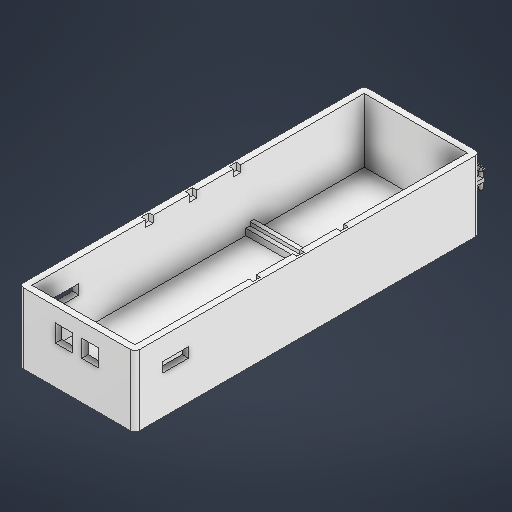
# Autodesk Inventor part: module_switch
Saved by Autodesk Inventor 2025.4 (Build 294407000, 407)
## iProperties
Created: 2025-09-07
Part Number: module_switch
Material: PC/ABS Plastic
Document SubType Name: Modeling
Designer: sam
Density: 1.1 g/cm^3
Appearance: Smooth - White
Author: sam
Autodesk Inventor part; units mm, degrees
ref_plane "YZ Plane" through (0, 0, 0) normal (1, 0, 0) x (0, 1, 0)
ref_plane "XZ Plane" through (0, 0, 0) normal (0, 1, 0) x (-1, 0, 0)
ref_plane "XY Plane" through (0, 0, 0) normal (0, 0, 1) x (1, 0, 0)
sketch "Sketch2" plane through (0, 0, 0) normal (0, 1, 0) x (-1, 0, 0)
  line L0 (-30.2, -84) -> (30.2, -84)
  line L1 (30.2, -84) -> (30.2, 84)
  line L2 (30.2, 84) -> (-30.2, 84)
  line L3 (-30.2, 84) -> (-30.2, -84)
  line L4 (-30.2, -84) -> (30.2, 84) construction
  line L5 (30.2, -84) -> (-30.2, 84) construction
  point P0 (0, 0)
  dimension "d0" = 60.4
  dimension "d1" = 168
  constraints: 12 end point, 2 midpoint, 2 parallel, 1 horizontal, 1 perpendicular
  measures "d0" distance of L2.end L1.end
  measures "d1" distance of L1.end L0.end
extrude "Extrusion1" add sketch "Sketch2" along normal blind 3
sketch "Sketch3" plane through (0, 3, 0) normal (0, 1, 0) x (1, 0, 0)
  line L0 (27.2, 81) -> (-27.2, 81)
  line L1 (-27.2, 81) -> (-27.2, -81)
  line L2 (-27.2, -81) -> (27.2, -81)
  line L3 (27.2, -81) -> (27.2, 81)
  line L4 (27.2, 81) -> (-27.2, -81) construction
  line L5 (-27.2, 81) -> (27.2, -81) construction
  line L6 (-30.2, 84) -> (-30.2, -84) projected
  line L7 (-30.2, -84) -> (30.2, -84) projected
  line L8 (24.2, 78) -> (-24.2, 78)
  line L9 (-24.2, 78) -> (-24.2, -78)
  line L10 (-24.2, -78) -> (24.2, -78)
  line L11 (24.2, -78) -> (24.2, 78)
  line L12 (24.2, 78) -> (-24.2, -78) construction
  line L13 (-24.2, 78) -> (24.2, -78) construction
  point P0 (0, 0)
  dimension "d4" = 3
  dimension "d5" = 3
  dimension "d6" = 3
  dimension "d7" = 3
  constraints: 24 end point, 4 midpoint, 4 parallel, 2 horizontal, 2 perpendicular
  measures "d4" distance between parallel lines of L6 L1
  measures "d5" distance between parallel lines of L7 L2
  measures "d6" distance between parallel lines of L2 L10
  measures "d7" distance between parallel lines of L1 L9
extrude "Extrusion2" add sketch "Sketch3" along normal blind 30
fillet "Fillet1" radius 2 8 edges at (27.2, 18, 81) (-27.2, 18, 81) (-30.2, 1.5, 84) (30.2, 1.5, 84) (27.2, 18, -81) (-27.2, 18, -81) (30.2, 1.5, -84) (-30.2, 1.5, -84)
sketch "Sketch10" plane through (0, 3, 0) normal (0, 1, 0) x (1, 0, 0)
  line L0 (24.2, 78) -> (-24.2, 78) projected
  line L1 (-24.2, 78) -> (-24.2, -78) projected
  line L2 (-24.2, -78) -> (24.2, -78) projected
  line L3 (24.2, -78) -> (24.2, 78) projected
  line L4 (-24.2, -78) -> (24.2, -78)
  line L5 (24.2, -78) -> (24.2, -73.8)
  line L6 (24.2, -73.8) -> (-24.2, -73.8)
  line L7 (-24.2, -73.8) -> (-24.2, -78)
  line L8 (-24.2, -73.8) -> (24.2, -73.8)
  line L9 (24.2, -73.8) -> (24.2, 22.4)
  line L10 (24.2, 22.4) -> (-24.2, 22.4)
  line L11 (-24.2, 22.4) -> (-24.2, -73.8)
  line L12 (-24.2, 22.4) -> (24.2, 22.4)
  line L13 (24.2, 22.4) -> (24.2, 26.4)
  line L14 (24.2, 26.4) -> (-24.2, 26.4)
  line L15 (-24.2, 26.4) -> (-24.2, 22.4)
  point P0 (0, 0)
  point P1 (-24.2, 26.4)
  point P2 (-24.2, 22.4)
  dimension "d90" = 4.2
  dimension "d91" = 96.2
  dimension "d92" = 4
  constraints: 24 end point, 6 parallel, 3 horizontal, 3 perpendicular, 3 point on line
  measures "d90" distance of L5.end L4.end
  measures "d91" distance of L9.end L8.end
  measures "d92" distance of L13.end L12.end
extrude "Extrusion9" add sketch "Sketch10" along normal blind 3 contours L3 L10 L1 L14 | L3 L2 L1 L6
sketch "Sketch11" plane through (0, 6, 0) normal (0, 1, 0) x (1, 0, 0)
  line L0 (-24.2, 22.4) -> (-24.2, 26.4) projected
  line L1 (-24.2, 22.4) -> (24.2, 22.4) projected
  line L2 (24.2, 26.4) -> (24.2, 22.4) projected
  line L3 (24.2, 26.4) -> (-24.2, 26.4) projected
  line L4 (-24.2, -78) -> (-24.2, -73.8) projected
  line L5 (24.2, -78) -> (-24.2, -78) projected
  line L6 (24.2, -73.8) -> (24.2, -78) projected
  line L7 (24.2, -73.8) -> (-24.2, -73.8) projected
  line L8 (24.2, 26.4) -> (-24.2, 26.4) projected
  line L9 (-24.2, 26.4) -> (24.2, 26.4)
  line L10 (24.2, 26.4) -> (24.2, 24.4)
  line L11 (24.2, 24.4) -> (-24.2, 24.4)
  line L12 (-24.2, 24.4) -> (-24.2, 26.4)
  line L13 (24.2, -73.8) -> (24.2, -78) projected
  line L14 (-24.2, -78) -> (24.2, -78)
  line L15 (24.2, -78) -> (24.2, -76)
  line L16 (24.2, -76) -> (-24.2, -76)
  line L17 (-24.2, -76) -> (-24.2, -78)
  point P0 (0, 0)
  point P1 (24.2, -72.6)
  point P2 (-24.2, -76)
  dimension "d95" = 2
  dimension "d120" = 2
  constraints: 16 end point, 4 parallel, 2 horizontal, 2 perpendicular, 2 point on line, 1 midpoint
  measures "d95" distance of L9.end L10.end
  measures "d120" distance of L15.end L14.end
extrude "Extrusion10" add sketch "Sketch11" along normal blind 1.6 contours L0 L3 L2 L11 | L4 L16 L6 L5
sketch "Sketch12" plane through (-25.2, 3, 81) normal (0, 0, 1) x (1, 0, 0)
  line L0 (-2, 30) -> (-2, 0) projected
  line L1 (0, 30) -> (50.4, 30) projected
  line L2 (-2, 30) -> (0, 30) projected
  line L3 (50.4, 30) -> (52.4, 30) projected
  line L4 (52.4, 0) -> (52.4, 30) projected
  line L5 (50.4, 0) -> (0, 0) projected
  line L6 (0, 0) -> (-2, 0) projected
  line L7 (52.4, 0) -> (50.4, 0) projected
  line L8 (15, 23.2) -> (23.06, 23.2)
  line L9 (23.06, 23.2) -> (23.06, 15)
  line L10 (23.06, 15) -> (15, 15)
  line L11 (15, 15) -> (15, 23.2)
  line L12 (27.34, 23.2) -> (35.4, 23.2)
  line L13 (35.4, 23.2) -> (35.4, 15)
  line L14 (35.4, 15) -> (27.34, 15)
  line L15 (27.34, 15) -> (27.34, 23.2)
  point P0 (25.2, -3)
  dimension "d116" = 8.06
  dimension "d117" = 8.2
  dimension "d118" = 15
  dimension "d119" = 17
  dimension "d121" = 8.06
  dimension "d122" = 8.2
  dimension "d123" = 15
  dimension "d124" = 17
  constraints: 16 end point, 4 parallel, 2 horizontal, 2 perpendicular
  measures "d116" distance of L9.end L10.end
  measures "d117" distance of L8.end L9.end
  measures "d118" distance between parallel lines of L5 L10
  measures "d119" distance between parallel lines of L0 L11
  measures "d121" distance of L13.end L14.end
  measures "d122" distance of L12.end L13.end
  measures "d123" distance between parallel lines of L5 L14
  measures "d124" distance between parallel lines of L4 L13
extrude "Extrusion11" cut sketch "Sketch12" against normal blind 3 contours L8 L9 L10 L11 | L12 L13 L14 L15
sketch "Sketch13" plane through (0, 3, 0) normal (0, 1, 0) x (1, 0, 0)
  arc A0 (-28.2, 84) -> (-30.2, 82) centre (-28.2, 82) ccw projected
  line L0 (-30.2, 82) -> (-30.2, -82) projected
  arc A1 (-30.2, -82) -> (-28.2, -84) centre (-28.2, -82) ccw projected
  line L1 (-28.2, -84) -> (28.2, -84) projected
  arc A2 (28.2, -84) -> (30.2, -82) centre (28.2, -82) ccw projected
  line L2 (30.2, -82) -> (30.2, 82) projected
  arc A3 (30.2, 82) -> (28.2, 84) centre (28.2, 82) ccw projected
  line L3 (28.2, 84) -> (-28.2, 84) projected
  line L4 (-25.2, 81) -> (25.2, 81) projected
  arc A4 (27.2, 79) -> (25.2, 81) centre (25.2, 79) ccw projected
  line L5 (27.2, 79) -> (27.2, -79) projected
  arc A5 (25.2, -81) -> (27.2, -79) centre (25.2, -79) ccw projected
  line L6 (25.2, -81) -> (-25.2, -81) projected
  arc A6 (-27.2, -79) -> (-25.2, -81) centre (-25.2, -79) ccw projected
  line L7 (-27.2, -79) -> (-27.2, 79) projected
  arc A7 (-25.2, 81) -> (-27.2, 79) centre (-25.2, 79) ccw projected
  point P0 (0, 0)
extrude "Extrusion12" cut sketch "Sketch13" against normal blind 3
sketch "Sketch14" plane through (25.2, 33, -81) normal (0, 0, -1) x (-1, 0, 0)
  line L0 (1, -10) -> (49.4, -10)
  line L1 (49.4, -10) -> (49.4, -19.6)
  line L2 (49.4, -19.6) -> (1, -19.6)
  line L3 (1, -19.6) -> (1, -10)
  line L4 (52.4, -33) -> (52.4, 0) projected
  line L5 (-2, 0) -> (-2, -33) projected
  line L6 (50.4, 0) -> (50.4, -33) projected
  line L7 (50.4, -33) -> (0, -33) projected
  point P0 (25.2, -33)
  point P1 (50.4, -16.5)
  point P2 (49.4, -14.8)
  dimension "d127" = 9.6
  dimension "d128" = 3
  dimension "d129" = 3
  dimension "d140" = 23
  constraints: 8 end point, 2 midpoint, 2 parallel, 1 horizontal, 1 perpendicular
  measures "d127" distance of L0.end L1.end
  measures "d128" distance between parallel lines of L4 L1
  measures "d129" distance between parallel lines of L5 L3
  measures "d140" distance between parallel lines of L7 L0
extrude "Extrusion13" add sketch "Sketch14" along normal blind 6
sketch "Sketch15" plane through (-24.2, 13.4, -81) normal (-1, 0, 0) x (0, 0, 1)
  line L0 (0, 9.6) -> (-6, 9.6) projected
  line L1 (0, 9.6) -> (-3.4, 9.6)
  line L2 (-3.4, 9.6) -> (-3.4, 6.6)
  line L3 (-3.4, 6.6) -> (0, 6.6)
  line L4 (0, 6.6) -> (0, 9.6)
  line L5 (0, 9.6) -> (0, 0) projected
  line L6 (0, 9.6) -> (-6, 9.6) projected
  line L7 (-6, 0) -> (-6, 9.6) projected
  line L8 (0, 0) -> (-6, 0) projected
  line L9 (0, 0) -> (-3.4, 0)
  line L10 (-3.4, 0) -> (-3.4, 3)
  line L11 (-3.4, 3) -> (0, 3)
  line L12 (0, 3) -> (0, 0)
  point P0 (81, -13.4)
  point P1 (-3.4, 0)
  dimension "d133" = 3.4
  dimension "d134" = 3
  dimension "d135" = 3.4
  dimension "d136" = 3
  constraints: 16 end point, 4 parallel, 2 horizontal, 2 perpendicular
  measures "d133" distance of L3.end L2.end
  measures "d134" distance of L2.end L1.end
  measures "d135" distance of L10.end L11.end
  measures "d136" distance of L9.end L10.end
extrude "Extrusion14" cut sketch "Sketch15" against normal up to surface (48.4 mm away) contours L4 L3 L2 L0 | L5 L8 L10 L11
fillet "Fillet8" radius 1 18 edges at (0, 23, -87) (0, 23, -84.4) (0, 13.4, -87) (0, 13.4, -84.4) (-24.2, 14.9, -84.4) (-24.2, 18.2, -87) (-24.2, 21.5, -84.4) (-24.2, 23, -85.7) (-24.2, 13.4, -85.7) (-24.2, 16.4, -82.7) (-24.2, 20, -82.7) (24.2, 20, -82.7) (24.2, 16.4, -82.7) (24.2, 14.9, -84.4) (24.2, 21.5, -84.4) (24.2, 23, -85.7) (24.2, 18.2, -87) (24.2, 13.4, -85.7)
sketch "Sketch16" plane through (-27.2, 0, -79) normal (-1, 0, 0) x (0, 0, 1)
  line L0 (147, 22.7) -> (134.9, 22.7)
  line L1 (134.9, 22.7) -> (134.9, 18)
  line L2 (134.9, 18) -> (147, 18)
  line L3 (147, 18) -> (147, 22.7)
  line L4 (160, 3) -> (160, 33) projected
  line L5 (152, 0) -> (0, 0) projected
  point P0 (79, 0)
  point P1 (154, 0)
  dimension "d141" = 12.1
  dimension "d142" = 4.7
  dimension "d143" = 13
  dimension "d144" = 18
  constraints: 8 end point, 2 parallel, 1 horizontal, 1 perpendicular, 1 other
  measures "d141" distance of L2.end L1.end
  measures "d142" distance of L1.end L0.end
  measures "d144" distance between parallel lines of L5 L2
extrude "Extrusion15" cut sketch "Sketch16" against normal through all
sketch "Sketch17" plane through (0, 33, 0) normal (0, 1, 0) x (1, 0, 0)
  arc A0 (-25.2, 81) -> (-27.2, 79) centre (-25.2, 79) ccw projected
  line L0 (-27.2, 79) -> (-27.2, -79) projected
  arc A1 (-27.2, -79) -> (-25.2, -81) centre (-25.2, -79) ccw projected
  line L1 (-25.2, -81) -> (25.2, -81) projected
  arc A2 (25.2, -81) -> (27.2, -79) centre (25.2, -79) ccw projected
  line L2 (27.2, -79) -> (27.2, 79) projected
  arc A3 (27.2, 79) -> (25.2, 81) centre (25.2, 79) ccw projected
  line L3 (25.2, 81) -> (-25.2, 81) projected
  line L4 (24.2, 78) -> (24.2, -78) projected
  line L5 (24.2, -78) -> (-24.2, -78) projected
  line L6 (-24.2, -78) -> (-24.2, 78) projected
  line L7 (-24.2, 78) -> (24.2, 78) projected
  line L8 (-26.2, 20) -> (-24.2, 20)
  line L9 (-24.2, 20) -> (-24.2, 16.6)
  line L10 (-24.2, 16.6) -> (-26.2, 16.6)
  line L11 (-26.2, 16.6) -> (-26.2, 20)
  line L12 (-24.2, -0.56) -> (-26.2, -0.56)
  line L13 (-26.2, -0.56) -> (-26.2, -3.96)
  line L14 (-26.2, -3.96) -> (-24.2, -3.96)
  line L15 (-24.2, -3.96) -> (-24.2, -0.56)
  line L16 (-24.2, 22.4) -> (-24.2, -73.8) projected
  line L17 (-24.2, -21.12) -> (-26.2, -21.12)
  line L18 (-26.2, -21.12) -> (-26.2, -24.52)
  line L19 (-26.2, -24.52) -> (-24.2, -24.52)
  line L20 (-24.2, -24.52) -> (-24.2, -21.12)
  line L21 (24.2, 20) -> (26.2, 20)
  line L22 (26.2, 20) -> (26.2, 16.6)
  line L23 (26.2, 16.6) -> (24.2, 16.6)
  line L24 (24.2, 16.6) -> (24.2, 20)
  line L25 (24.2, -0.56) -> (26.2, -0.56)
  line L26 (26.2, -0.56) -> (26.2, -3.96)
  line L27 (26.2, -3.96) -> (24.2, -3.96)
  line L28 (24.2, -3.96) -> (24.2, -0.56)
  line L29 (24.2, -21.12) -> (26.2, -21.12)
  line L30 (26.2, -21.12) -> (26.2, -24.52)
  line L31 (26.2, -24.52) -> (24.2, -24.52)
  line L32 (24.2, -24.52) -> (24.2, -21.12)
  point P0 (0, 0)
  point P1 (-24.2, 16.6)
  point P2 (24.2, 16.6)
  point P3 (24.2, -3.96)
  point P4 (24.2, -24.52)
  point P5 (-24.2, -24.52)
  point P6 (-24.2, -21.12)
  point P7 (-24.2, -3.96)
  dimension "d147" = 2
  dimension "d148" = 3.4
  dimension "d149" = 61
  dimension "d150" = 0
  dimension "d153" = 2
  dimension "d154" = 3.4
  dimension "d155" = 20.56
  dimension "d156" = 2
  dimension "d157" = 3.4
  dimension "d158" = 20.56
  dimension "d159" = 2
  dimension "d160" = 3.4
  dimension "d161" = 2
  dimension "d162" = 3.4
  dimension "d163" = 2
  dimension "d164" = 3.4
  dimension "d165" = 20.56
  dimension "d166" = 20.56
  dimension "d167" = 61
  constraints: 48 end point, 12 parallel, 6 horizontal, 6 perpendicular, 5 point on line
  measures "d147" distance of L9.end L10.end
  measures "d148" distance of L8.end L9.end
  measures "d149" distance between parallel lines of L3 L8
  measures "d150" distance between parallel lines of L6 L9
  measures "d153" distance of L14.end L13.end
  measures "d154" distance of L13.end L12.end
  measures "d155" distance between parallel lines of L12 L8
  measures "d156" distance of L19.end L18.end
  measures "d157" distance of L18.end L17.end
  measures "d158" distance between parallel lines of L12 L17
  measures "d159" distance of L22.end L23.end
  measures "d160" distance of L21.end L22.end
  measures "d161" distance of L26.end L27.end
  measures "d162" distance of L25.end L26.end
  measures "d163" distance of L30.end L31.end
  measures "d164" distance of L29.end L30.end
  measures "d165" distance between parallel lines of L25 L29
  measures "d166" distance between parallel lines of L21 L25
  measures "d167" distance between parallel lines of L3 L21
extrude "Extrusion16" cut sketch "Sketch17" against normal blind 3.2 contours L21 L22 L23 L4 | L25 L26 L27 L4 | L6 L10 L11 L8 | L29 L30 L31 L4 | L6 L14 L13 L12 | L6 L19 L18 L17
equation "\"d167\" = d149"
body "Solid1"
